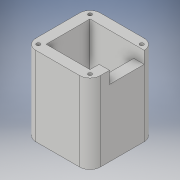
# Autodesk Inventor part: 000.207 - Поддержка центра
Saved by Autodesk Inventor 2019 (Build 230136000, 136)
## iProperties
Created: 2020-03-06
Part Number: 000.207 - Поддержка центра
Material: Типовые
Document SubType Name: Modeling
Designer: Петров Иван
Density: 1 g/cm^3
Appearance: По умолчанию
Author: Петров Иван
Autodesk Inventor part; units mm, degrees
ref_plane "YZ Plane" through (0, 0, 0) normal (1, 0, 0) x (0, 1, 0)
ref_plane "XZ Plane" through (0, 0, 0) normal (0, 1, 0) x (-1, 0, 0)
ref_plane "XY Plane" through (0, 0, 0) normal (0, 0, 1) x (1, 0, 0)
sketch "Эскиз1" plane through (0, 0, 0) normal (0, 1, 0) x (-1, 0, 0)
  arc A0 (-18, 26.5) -> (-26.5, 18) centre (-18, 18) ccw
  line L0 (-26.5, -18) -> (-26.5, 18)
  arc A1 (-26.5, -18) -> (-18, -26.5) centre (-18, -18) ccw
  line L1 (18, -26.5) -> (-18, -26.5)
  arc A2 (18, -26.5) -> (26.5, -18) centre (18, -18) ccw
  line L2 (26.5, 18) -> (26.5, -18)
  arc A3 (26.5, 18) -> (18, 26.5) centre (18, 18) ccw
  line L3 (-18, 26.5) -> (18, 26.5)
  circle A4 centre (-21.2132, 21.2132) radius 1.5
  circle A5 centre (-21.2132, -21.2132) radius 1.5
  circle A6 centre (21.2132, -21.2132) radius 1.5
  circle A7 centre (21.2132, 21.2132) radius 1.5
  line L4 (18, 18) -> (-18, 18)
  line L5 (-18, 18) -> (-18, -18)
  line L6 (-18, -18) -> (18, -18)
  line L7 (18, -18) -> (18, 18)
  point P0 (0, 0)
  point P1 (0, 0)
  constraints: 16 end point, 8 centre point, 8 point on circle, 2 parallel, 1 horizontal, 1 perpendicular
extrude "Выдавливание1" add sketch "Эскиз1" along normal blind 65
sketch "Эскиз5" plane through (-18, 0, 26.5) normal (0, 0, 1) x (1, 0, 0)
  line L0 (-33.8256, 77.7148) -> (54.9741, 77.7148)
  line L1 (54.9741, 77.7148) -> (54.9741, -14.3336)
  line L2 (54.9741, -14.3336) -> (-33.8256, -14.3336)
  line L3 (-33.8256, -14.3336) -> (-33.8256, 77.7148)
  point P0 (18, 0)
  constraints: 8 end point, 2 parallel, 1 horizontal, 1 perpendicular
extrude "Выдавливание5" [suppressed]
sketch "Эскиз6" plane through (0, 65, 0) normal (0, 1, 0) x (1, 0, 0)
  line L0 (26.5, -18) -> (26.5, 18) projected
  line L1 (18, 18) -> (18, -18) projected
  line L2 (26.5, 18) -> (18, 18)
  line L3 (18, 18) -> (18, -10.5)
  line L4 (18, -10.5) -> (26.5, -10.5)
  line L5 (26.5, -10.5) -> (26.5, 18)
  point P0 (0, 0)
  constraints: 8 end point, 2 parallel, 1 horizontal, 1 perpendicular
extrude "Выдавливание6" cut sketch "Эскиз6" against normal blind 10
